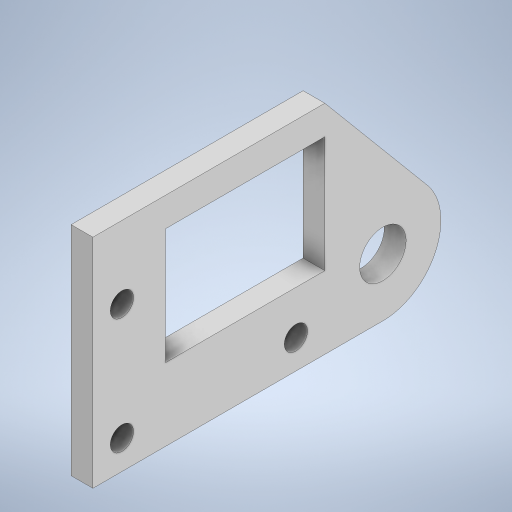
# Autodesk Inventor part: battery_cover_setter_joint
Saved by Autodesk Inventor 2024.1 (Build 281209000, 209)
## iProperties
Created: 2024-10-11
Part Number: battery_cover_setter_joint
Material: 一般
Document SubType Name: Sheet Metal
Designer: hibik
Density: 1 g/cm^3
Sheet Metal Rule: Default_mm
Appearance: 既定
Flat Pattern Width: 1.5 cm
Flat Pattern Length: 2.4 cm
Flat Pattern Area: 3.6 cm^2
Sheet Metal Width: 15.000 mm
Sheet Metal Length: 24.000 mm
Sheet Metal Area: 360.000 mm^2
Author: hibik
Autodesk Inventor part; units mm, degrees
ref_plane "YZ Plane" through (0, 0, 0) normal (1, 0, 0) x (0, 1, 0)
ref_plane "XZ Plane" through (0, 0, 0) normal (0, 1, 0) x (-1, 0, 0)
ref_plane "XY Plane" through (0, 0, 0) normal (0, 0, 1) x (1, 0, 0)
sketch "スケッチ1" plane through (0, 0, 0) normal (1, 0, 0) x (0, 1, 0)
  line L0 (0, 0) -> (15, 0)
  line L1 (15, 0) -> (15, -16)
  line L2 (15, -16) -> (0, -16)
  line L3 (0, -16) -> (0, 0)
  circle A0 centre (4, -20) radius 4
  circle A1 centre (4, -20) radius 1.6
  line L4 (15, -16) -> (6.5693, -23.0657)
  line L5 (0, -20) -> (0, -16)
  dimension "d0" = 15
  dimension "d2" = 3.2
  dimension "d3" = 8
  dimension "d5" = 20
  measures "d0" distance of L1.end L2.end
  measures "d2" diameter of A1
  measures "d3" diameter of A0
  measures "d5" distance from line of L0 A0.centre
extrude "プレート1" add sketch "スケッチ1" along normal blind 1.5
sketch "スケッチ2" plane through (1.5, 0, 0) normal (1, 0, 0) x (0, 0, -1)
  circle A0 centre (2, 10) radius 0.8 projected
  circle A1 centre (2, 2) radius 0.8 projected
  circle A2 centre (20, 4) radius 1.6 projected
  line L0 (0, 15) -> (16, 15) projected
  line L1 (0, 0) -> (0, 15) projected
  line L2 (20, 0) -> (0, 0) projected
  arc A3 (20, 0) -> (23.0657, 6.5693) centre (20, 4) ccw projected
  line L3 (16, 15) -> (23.0657, 6.5693) projected
  circle A4 centre (14, 2) radius 0.8 projected
  line L4 (5, 13) -> (16, 13)
  line L5 (16, 13) -> (16, 5)
  line L6 (16, 5) -> (5, 5)
  line L7 (5, 5) -> (5, 13)
  dimension "d8" = 2
  dimension "d9" = 3
  dimension "d10" = 3
  constraints: 8 end point, 2 parallel, 1 horizontal, 1 perpendicular, 1 point on line
  measures "d8" distance between parallel lines of L0 L4
  measures "d9" distance from line of A0.centre L7
  measures "d10" distance from line of A4.centre L6
extrude "切り取り1" cut sketch "スケッチ2" against normal blind 1.5 contours A0 | A1 | A4 | L4 L5 L6 L7
equation "\"d6\" = Thickness"
equation "\"d4\" = Thickness"
equation "\"BendRadius\" = Thickness"
equation "\"BendReliefWidth\" = Thickness"
equation "\"BendReliefDepth\" = 0.5 * Thickness"
equation "\"CornerReliefSize\" = 4 * Thickness"
equation "\"MinimumRemnant\" = 2 * Thickness"
equation "\"TransitionRadius\" = BendRadius"
equation "\"JacobiRadiusSize\" = BendRadius"
equation "\"GapSize\" = Thickness"
equation "\"Thickness\" = 1.5"
